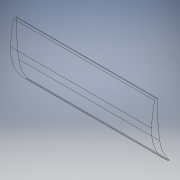
# Autodesk Inventor part: cover_re
Saved by Autodesk Inventor 2018.1 (Build 221171000, 171)
## iProperties
Created: 2017-10-27
Part Number: cover_re
Material: CFRP
Document SubType Name: Modeling
Designer: kuwano
Density: 1.43 g/cm^3
Appearance: カーボンファイバー
Mass: 1331.35 g
Surface Area: 18629.9 cm^2
Volume: 931.013 cm^3
Author: kuwano
Autodesk Inventor part; units mm, degrees
ref_plane "YZ Plane" through (0, 0, 0) normal (1, 0, 0) x (0, 1, 0)
ref_plane "XZ Plane" through (0, 0, 0) normal (0, 1, 0) x (-1, 0, 0)
ref_plane "XY Plane" through (0, 0, 0) normal (0, 0, 1) x (1, 0, 0)
sketch "スケッチ1" plane through (0, 0, 0) normal (1, 0, 0) x (0, 1, 0)
  line L0 (0, 250) -> (88.1635, -250)
  line L1 (0, 355.3665) -> (0, -371.5339) projected
  arc A0 (0, 250) -> (10.0651, -90) centre (1573.0305, 126.4177) ccw
  arc A1 (10.0651, -90) -> (88.1635, -250) centre (293.3792, -50.7706) ccw
  arc A2 (0, 250) -> (-44.6969, 9.8272) centre (854.2727, -33.2282) ccw
  arc A3 (-44.6969, 9.8272) -> (88.1635, -250) centre (248.3498, -4.208) ccw
  point P0 (0, 0)
  dimension "d0" = 10
  dimension "d1" = 500
  dimension "d4" = 250
  dimension "d10" = 1577.8776
  dimension "d11" = 286.0172
  dimension "d12" = 160
  dimension "d13" = 900
  constraints: 8 point on circle, 4 centre point, 2 end point, 2 tangent, 1 point on line
  measures "d0" angle of L1 L0
  measures "d1" vertical distance of L0.end L0.start
  measures "d4" distance of point (0, 0) L0.start
  measures "d10" radius of A0
  measures "d11" radius of A1
  measures "d12" vertical distance of L0.end A0.end
  measures "d13" radius of A2
extrude "押し出し2" add sketch "スケッチ1" along normal mid plane 950 contours A0 L1 A3 A2 | A3 L1 A0 A1
fillet "フィレット3" radius 10 1 edges at (0, 0, 250)
fillet "フィレット3" radius 2 1 edges at (0, 88.1635, -250)
